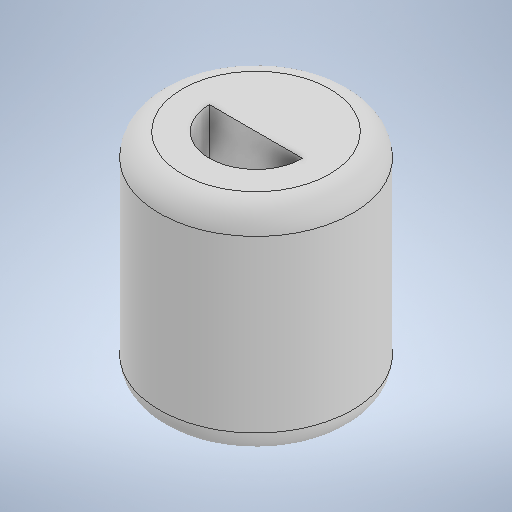
# Autodesk Inventor part: Connector 001
Saved by Autodesk Inventor 2025 (Build 290162000, 162)
## iProperties
Created: 2024-04-11
Part Number: Connector 001
Material: Generisch
Document SubType Name: Modeling
Designer: noahm
Density: 1 g/cm^3
Appearance: Vorgabe
Author: noahm
Autodesk Inventor part; units mm, degrees
ref_plane "YZ Plane" through (0, 0, 0) normal (1, 0, 0) x (0, 1, 0)
ref_plane "XZ Plane" through (0, 0, 0) normal (0, 1, 0) x (-1, 0, 0)
ref_plane "XY Plane" through (0, 0, 0) normal (0, 0, 1) x (1, 0, 0)
sketch "Skizze1" plane through (0, 0, 0) normal (0, 0, 1) x (1, 0, 0)
  circle A0 centre (0, 0) radius 8.5
  dimension "d0" = 17
  constraints: 1 centre point, 1 coincident
  measures "d0" diameter of A0
extrude "Extrusion1" add sketch "Skizze1" along normal blind 19
fillet "Rundung1" radius 2 2 edges at (-8.5, 0, 19) (-8.5, 0, 0)
sketch "Skizze2" plane through (0, 0, 19) normal (0, 0, 1) x (1, 0, 0)
  arc A0 (-4.1, 0) -> (4.1, 0) centre (0, 0) ccw
  line L0 (-4.1, 0) -> (4.1, 0)
  dimension "d4" = 8.2
  constraints: 2 end point, 2 point on circle, 1 centre point, 1 coincident, 1 horizontal
  measures "d4" diameter of A0
extrude "Extrusion2" cut sketch "Skizze2" against normal blind 8.2
sketch "Skizze3" plane through (0, 0, 0) normal (0, 0, -1) x (-1, 0, 0)
  arc A0 (1.462, -2.15) -> (-1.462, -2.15) centre (0, 0) ccw
  line L0 (-1.462, -2.15) -> (1.462, -2.15)
  point P0 (0, -2.15)
  dimension "d8" = 5.2
  constraints: 2 end point, 2 point on circle, 1 centre point, 1 coincident, 1 midpoint
  measures "d8" diameter of A0
extrude "Extrusion3" cut sketch "Skizze3" against normal blind 8.2
